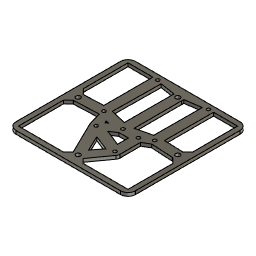
Base_v1_boitier (Autodesk Fusion 360 design; units mm, degrees)
Autodesk Fusion 360 part; units mm, degrees
note: some values were not read from the file. Set by a fixed rule: which sketch regions a step uses.
sketch "Sketch1" plane through (0, 0, 0) normal (0, 0, 1) x (1, 0, 0)
  line L0 (-52.5, 60) -> (52.5, 60)
  line L1 (60, 52.5) -> (60, -52.5)
  line L2 (52.5, -60) -> (-52.5, -60)
  line L3 (-60, -52.5) -> (-60, 52.5)
  line L4 (0, 0) -> (0, 50)
  line L5 (0, 0) -> (-50, 0)
  line L6 (0, 0) -> (50, 0)
  line L7 (0, 0) -> (0, -50)
  circle A0 centre (0, 50) radius 2.25
  circle A1 centre (-50, 0) radius 2.25
  circle A2 centre (50, 0) radius 2.25
  circle A3 centre (0, -50) radius 2.25
  arc A4 (-52.5, 60) -> (-60, 52.5) centre (-52.5, 52.5) ccw
  arc A5 (60, 52.5) -> (52.5, 60) centre (52.5, 52.5) ccw
  arc A6 (52.5, -60) -> (60, -52.5) centre (52.5, -52.5) ccw
  arc A7 (-60, -52.5) -> (-52.5, -60) centre (-52.5, -52.5) ccw
  point P0 (-60, 60)
  point P1 (60, 60)
  point P2 (-60, -60)
  dimension "d1" = 120
  dimension "d2" = 120
  dimension "d3" = 50
  dimension "d4" = 50
  dimension "d5" = 50
  dimension "d6" = 4.5
  dimension "d7" = 4.5
  dimension "d8" = 4.5
  dimension "d9" = 4.5
  dimension "d10" = 7.5
  constraint horizontal L0
  constraint vertical L1
  constraint horizontal L2
  constraint vertical L3
  constraint coincident L4.start L5.start
  constraint vertical L4
  constraint perpendicular L4 L5
  constraint perpendicular L4 L6
  constraint perpendicular L5 L7
  constraint coincident L4.end A0.centre
  constraint coincident L5.end A1.centre
  constraint coincident L6.end A2.centre
  constraint coincident L7.end A3.centre
  constraint coincident P0 L0
  constraint coincident P0 L3
  constraint tangent L0 A4
  constraint tangent L3 A4
  constraint coincident P1 L0
  constraint coincident P1 L1
  constraint tangent L0 A5
  constraint tangent L1 A5
  constraint equal A4 A5
  constraint tangent L1 A6
  constraint tangent L2 A6
  constraint equal A4 A6
  constraint coincident P2 L2
  constraint coincident P2 L3
  constraint tangent L2 A7
  constraint tangent L3 A7
  constraint equal A4 A7
  measures "d1" distance of P0 P1
  measures "d2" distance of P0 P2
  measures "d3" distance of L4.start L4.end
  measures "d4" distance of L4.start L5.end
  measures "d5" distance of L4.start L6.end
  measures "d6" diameter of A0
  measures "d7" diameter of A1
  measures "d8" diameter of A2
  measures "d9" diameter of A3
  measures "d10" radius of A4
extrude "Extrude1" add sketch "Sketch1" along normal blind 3.3
sketch "Sketch2" plane through (0, 0, 3.3) normal (0, 0, 1) x (-1, 0, 0)
  circle A0 centre (0, -50) radius 2.25
  circle A1 centre (50, 0) radius 2.25
  circle A2 centre (0, 50) radius 2.25
  circle A3 centre (-50, 0) radius 2.25
  arc A4 (52.5, -60) -> (60, -52.5) centre (52.5, -52.5) ccw
  line L0 (60, -52.5) -> (60, 52.5)
  arc A5 (60, 52.5) -> (52.5, 60) centre (52.5, 52.5) ccw
  line L1 (52.5, 60) -> (-52.5, 60)
  arc A6 (-52.5, 60) -> (-60, 52.5) centre (-52.5, 52.5) ccw
  line L2 (-60, 52.5) -> (-60, -52.5)
  arc A7 (-60, -52.5) -> (-52.5, -60) centre (-52.5, -52.5) ccw
  line L3 (-52.5, -60) -> (52.5, -60)
  line L4 (25.0941, -54.9843) -> (-25.9059, -54.9843)
  line L5 (-25.9059, -54.9843) -> (-25.9059, -0.9843)
  line L6 (-25.9059, -0.9843) -> (25.0941, -0.9843)
  line L7 (25.0941, -0.9843) -> (25.0941, -54.9843)
  circle A8 centre (25.0941, -54.9843) radius 1.7
  circle A9 centre (-25.9059, -54.9843) radius 1.7
  circle A10 centre (-25.9059, -0.9843) radius 1.7
  circle A11 centre (25.0941, -0.9843) radius 1.7
  line L8 (0, 5) -> (-15.5, 5)
  circle A12 centre (-15.5, 5) radius 1.7
  circle A13 centre (0, 5) radius 1.7
  line L9 (-15.5, 5) -> (-15.5, 28.5)
  circle A14 centre (-15.5, 28.5) radius 1.7
  line L10 (0, 5) -> (16.2982, 15.7059)
  line L11 (0, 5) -> (19.5, 5) construction
  circle A15 centre (16.2982, 15.7059) radius 1.7
  dimension "d13" = 51
  dimension "d14" = 54
  dimension "d15" = 3.4
  dimension "d16" = 3.4
  dimension "d17" = 3.4
  dimension "d18" = 3.4
  dimension "d19" = 15.5
  dimension "d20" = 3.4
  dimension "d21" = 3.4
  dimension "d22" = 23.5
  dimension "d23" = 3.4
  dimension "d24" = 19.5
  dimension "d25" = 33.3
  dimension "d26" = 3.4
  constraint horizontal L4
  constraint vertical L5
  constraint horizontal L6
  constraint vertical L7
  constraint coincident L4.start L7.end
  constraint coincident L4.end L5.start
  constraint coincident L5.end L6.start
  constraint coincident L6.end L7.start
  constraint horizontal L8
  constraint coincident L8.end A12.centre
  constraint coincident L8.start A13.centre
  constraint perpendicular L8 L9
  constraint coincident L9.end A14.centre
  constraint horizontal L11
  constraint coincident L10.end A15.centre
  measures "d13" distance of L4.start L4.end
  measures "d14" distance of L4.start L6.end
  measures "d15" diameter of A8
  measures "d16" diameter of A9
  measures "d17" diameter of A10
  measures "d18" diameter of A11
  measures "d19" distance of L8.start L8.end
  measures "d20" diameter of A12
  measures "d21" diameter of A13
  measures "d22" distance of L8.end L9.end
  measures "d23" diameter of A14
  measures "d24" distance of L8.start L10.end
  measures "d25" angle of L10 L11
  measures "d26" diameter of A15
extrude "Extrude2" cut sketch "Sketch2" against normal blind 5 contours L4 L5 A9 | L4 L5 A9 | L4 L7 A8 | L4 L7 A8 | L5 L6 A10 | L5 L6 A10 | L6 L7 A11 | L6 L7 A11 | L8 A12 L9 | L8 A12 L9 | L8 A13 L10 | L8 A13 L10 | A14 | A15
sketch "Sketch3" plane through (0, 0, 3.3) normal (0, 0, 1) x (-1, 0, 0)
  circle A0 centre (-15.5, 28.5) radius 1.7
  circle A1 centre (25.0941, -0.9843) radius 1.7
  circle A2 centre (16.2982, 15.7059) radius 1.7
  circle A3 centre (-25.9059, -0.9843) radius 1.7
  circle A4 centre (-15.5, 5) radius 1.7
  circle A5 centre (25.0941, -54.9843) radius 1.7
  circle A6 centre (0, 5) radius 1.7
  circle A7 centre (-25.9059, -54.9843) radius 1.7
  circle A8 centre (0, -50) radius 2.25
  circle A9 centre (50, 0) radius 2.25
  circle A10 centre (0, 50) radius 2.25
  circle A11 centre (-50, 0) radius 2.25
  arc A12 (52.5, -60) -> (60, -52.5) centre (52.5, -52.5) ccw
  line L0 (60, -52.5) -> (60, 52.5)
  arc A13 (60, 52.5) -> (52.5, 60) centre (52.5, 52.5) ccw
  line L1 (52.5, 60) -> (-52.5, 60)
  arc A14 (-52.5, 60) -> (-60, 52.5) centre (-52.5, 52.5) ccw
  line L2 (-60, 52.5) -> (-60, -52.5)
  arc A15 (-60, -52.5) -> (-52.5, -60) centre (-52.5, -52.5) ccw
  line L3 (-52.5, -60) -> (52.5, -60)
  line L4 (55, -55) -> (-55, -55)
  line L5 (-55, -55) -> (-55, 55)
  line L6 (-55, 55) -> (55, 55)
  line L7 (55, 55) -> (55, -55)
  circle A16 centre (25.0941, -54.9843) radius 5
  circle A17 centre (0, -50) radius 5
  circle A18 centre (-25.9059, -54.9843) radius 5
  circle A19 centre (50, 0) radius 5
  circle A20 centre (25.0941, -0.9843) radius 5
  circle A21 centre (0, 5) radius 5
  circle A22 centre (-25.9059, -0.9843) radius 5
  circle A23 centre (-15.5, 5) radius 5
  circle A24 centre (-50, 0) radius 5
  circle A25 centre (16.2982, 15.7059) radius 5
  circle A26 centre (-15.5, 28.5) radius 5
  circle A27 centre (0, 50) radius 5
  line L8 (20.3339, -53.4544) -> (4.8903, -51.0416)
  line L9 (20.3339, -53.4544) -> (-21.1457, -53.4544)
  line L10 (4.8903, -51.0416) -> (-4.8903, -51.0416)
  line L11 (-21.1457, -53.4544) -> (-4.8903, -51.0416)
  line L12 (55, -10.2174) -> (49.9843, -5)
  line L13 (50, 5) -> (55, 9.8066)
  line L14 (5, 50) -> (10, 55)
  line L15 (-5, 50) -> (-10, 55)
  line L16 (-50, -5) -> (-55, -10)
  line L17 (-50, 5) -> (-55, 10)
  line L18 (49.9843, -5) -> (25.2925, -5.9804)
  line L19 (50, 5) -> (24.8975, 4.0118)
  line L20 (24.8975, 4.0118) -> (21.1002, 17.0992)
  line L21 (20.7089, -3.3864) -> (11.875, 13.3747)
  line L22 (22.8445, -5.4496) -> (-1.1332, 0.1301)
  line L23 (24.8975, 4.0118) -> (1.1968, 9.8547)
  line L24 (13.0471, 19.5047) -> (-2.7362, 9.1849)
  line L25 (19.3563, 11.7501) -> (3.3352, 1.2749)
  line L26 (30.0941, -55) -> (30.0941, -0.9843)
  line L27 (20.0942, -55) -> (20.7089, -3.3864)
  line L28 (4.8903, -51.0416) -> (5, 4.9902)
  line L29 (-4.8903, -51.0416) -> (-5, 4.9902)
  line L30 (-21.1457, -53.4544) -> (-20.9059, -1.0072)
  line L31 (-30.9058, -55) -> (-30.9059, -0.9843)
  line L32 (0, 0) -> (-24.7559, -5.8503)
  line L33 (-1.1332, 10.233) -> (-15.5808, 9.9993)
  line L34 (-27.5548, 3.736) -> (-18.0263, 9.3148)
  line L35 (-50, 5) -> (-27.5548, 3.736)
  line L36 (-50, -5) -> (-26.1108, -5.9801)
  line L37 (-15.2954, 33.4958) -> (18.1272, 20.3594)
  line L38 (14.7074, 10.9658) -> (-17.3652, 23.8609)
  line L39 (-10.554, 5.7326) -> (-10.5, 28.4881)
  line L40 (-20.4003, 4.0065) -> (-20.5, 28.4796)
  line L41 (-10.5, 28.4881) -> (3.9361, 46.9166)
  line L42 (-19.4676, 31.5427) -> (-4.0561, 52.9237)
  line L43 (21.1002, 17.0992) -> (5, 50)
  line L44 (11.875, 13.3747) -> (-4.5157, 47.8533)
  dimension "d29" = 10
  dimension "d30" = 10
  dimension "d31" = 10
  dimension "d32" = 10
  dimension "d33" = 10
  dimension "d34" = 10
  dimension "d35" = 10
  dimension "d36" = 10
  dimension "d37" = 10
  dimension "d38" = 10
  dimension "d39" = 10
  dimension "d40" = 10
  constraint horizontal L4
  constraint vertical L5
  constraint horizontal L6
  constraint vertical L7
  constraint concentric A5 A16
  constraint concentric A8 A17
  constraint concentric A7 A18
  constraint concentric A9 A19
  constraint concentric A1 A20
  constraint concentric A6 A21
  constraint concentric A3 A22
  constraint concentric A4 A23
  constraint concentric A11 A24
  constraint concentric A2 A25
  constraint concentric A0 A26
  constraint concentric A10 A27
  constraint coincident A16 L8.start
  constraint coincident A17 L8.end
  constraint coincident A18 L9.end
  constraint parallel L4 L9
  constraint coincident A17 L10.end
  constraint parallel L9 L10
  constraint coincident L7 L12.start
  constraint coincident A19 L12.end
  constraint coincident A19 L13.start
  constraint perpendicular L12 L13
  constraint coincident A27 L14.start
  constraint coincident L6 L14.end
  constraint coincident A27 L15.start
  constraint coincident L6 L15.end
  constraint perpendicular L14 L15
  constraint coincident A24 L16.start
  constraint coincident L5 L16.end
  constraint perpendicular L15 L16
  constraint coincident A24 L17.start
  constraint coincident L5 L17.end
  constraint perpendicular L16 L17
  constraint coincident A20 L18.end
  constraint tangent A20 L18
  constraint coincident A20 L19.end
  constraint tangent A20 L19
  constraint coincident A25 L20.end
  constraint tangent A25 L20
  constraint coincident A20 L21.start
  constraint coincident A25 L21.end
  constraint tangent A25 L21
  constraint coincident A20 L22.start
  constraint coincident A21 L22.end
  constraint tangent A21 L22
  constraint coincident A21 L23.end
  constraint tangent A21 L23
  constraint coincident A25 L24.start
  constraint coincident A21 L24.end
  constraint tangent A21 L24
  constraint coincident A25 L25.start
  constraint coincident A21 L25.end
  constraint parallel L24 L25
  constraint coincident A16 L26.start
  constraint coincident L4 L26.start
  constraint coincident A20 L26.end
  constraint tangent A20 L26
  constraint coincident A16 L27.start
  constraint coincident L4 L27.start
  constraint coincident A21 L28.end
  constraint tangent A21 L28
  constraint coincident A21 L29.end
  constraint tangent A21 L29
  constraint coincident A22 L30.end
  constraint tangent A22 L30
  constraint coincident L4 L31.start
  constraint coincident A18 L31.start
  constraint coincident A22 L31.end
  constraint tangent A22 L31
  constraint coincident L32.start origin
  constraint coincident A22 L32.end
  constraint tangent A22 L32
  constraint coincident L24 L33.start
  constraint coincident A23 L33.end
  constraint tangent A23 L33
  constraint coincident A22 L34.start
  constraint coincident A23 L34.end
  constraint tangent A23 L34
  constraint coincident A22 L36.end
  constraint tangent A22 L36
  constraint coincident A26 L37.start
  constraint coincident A25 L37.end
  constraint tangent A25 L37
  constraint coincident A25 L38.start
  constraint coincident A26 L38.end
  constraint tangent A26 L38
  constraint coincident A23 L39.start
  constraint coincident A26 L39.end
  constraint tangent A26 L39
  constraint coincident A23 L40.start
  constraint coincident A26 L40.end
  constraint tangent A26 L40
  constraint coincident A27 L41.end
  constraint tangent A27 L41
  constraint coincident A26 L42.start
  constraint coincident A27 L42.end
  constraint tangent A27 L42
  constraint coincident A27 L44.end
  constraint tangent A27 L44
  measures "d29" diameter of A16
  measures "d30" diameter of A17
  measures "d31" diameter of A18
  measures "d32" diameter of A19
  measures "d33" diameter of A20
  measures "d34" diameter of A21
  measures "d35" diameter of A22
  measures "d36" diameter of A23
  measures "d37" diameter of A24
  measures "d38" diameter of A25
  measures "d39" diameter of A26
  measures "d40" diameter of A27
extrude "Extrude3" cut sketch "Sketch3" against normal blind 5 contours L4 L7 A16 L12 L18 L26 | L4 L5 L16 L31 L36 | A17 L8 L22 L27 L28 | L6 L7 A25 L13 L14 L19 L20 L43 | A17 L11 L29 L30 L32 | L21 L23 L25 | L5 L6 A24 A26 L15 L17 L34 L35 L40 L42 | L24 L33 L38 L39 | L37 L41 L44
sketch "Sketch4" plane through (0, 0, 0) normal (0, 0, 1) x (1, 0, 0)
